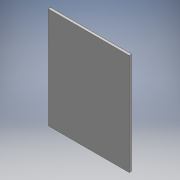
# Autodesk Inventor part: plytka2
Saved by Autodesk Inventor 2016 (Build 200138000, 138)
## iProperties
Created: 2015-11-09
Part Number: plytka2
Material: Ogólny
Document SubType Name: Modeling
Designer: Mrianura
Density: 1 g/cm^3
Appearance: Domyślna
Author: Mrianura
Autodesk Inventor part; units mm, degrees
ref_plane "YZ Plane" through (0, 0, 0) normal (1, 0, 0) x (0, 1, 0)
ref_plane "XZ Plane" through (0, 0, 0) normal (0, 1, 0) x (-1, 0, 0)
ref_plane "XY Plane" through (0, 0, 0) normal (0, 0, 1) x (1, 0, 0)
sketch "Szkic1" plane through (0, 0, 0) normal (0, 1, 0) x (-1, 0, 0)
  line L0 (0, 0) -> (0, -86)
  line L1 (0, -86) -> (68.7, -86)
  line L2 (68.7, -86) -> (68.7, 0)
  line L3 (68.7, 0) -> (0, 0)
  dimension "d0" = 86
  dimension "d1" = 68.7
  constraints: 8 end point, 3 perpendicular, 1 vertical
  measures "d0" distance of L0.start L0.end
  measures "d1" distance of L0.end L1.end
extrude "Wyciągnięcie proste1" add sketch "Szkic1" along normal blind 2
